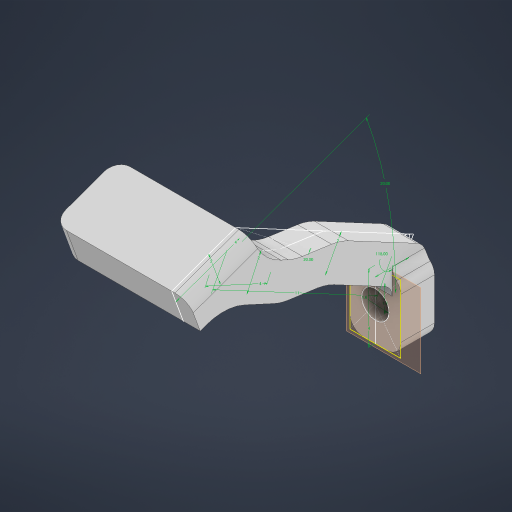
# Autodesk Inventor part: battery-stopper-1
Saved by Autodesk Inventor 2023.5 (Build 275446000, 446)
## iProperties
Created: 2025-02-09
Part Number: battery-stopper-1
Material: 一般
Document SubType Name: Modeling
Designer: IshiiLabHonda
Density: 1 g/cm^3
Appearance: 既定
Author: IshiiLabHonda
Autodesk Inventor part; units mm, degrees
ref_plane "YZ Plane" through (0, 0, 0) normal (1, 0, 0) x (0, 1, 0)
ref_plane "XZ Plane" through (0, 0, 0) normal (0, 1, 0) x (-1, 0, 0)
ref_plane "XY Plane" through (0, 0, 0) normal (0, 0, 1) x (1, 0, 0)
sketch "スケッチ5" plane through (0, 0, 0) normal (1, 0, 0) x (0, 1, 0)
  line L0 (0, 0) -> (0, 1.293622) construction
  line L1 (0, 0) -> (-1.333849, 0) construction
  line L2 (2, 2) -> (-2, 2)
  line L3 (-2, 2) -> (-2, 0)
  line L4 (-2, 0) -> (2, 0)
  line L5 (2, 0) -> (2, 2)
  line L6 (0.8, 2) -> (0.8, 0)
  line L7 (-0.8, 2) -> (-0.8, 0)
  line L8 (-2, 1) -> (2, 1) construction
  line L9 (2, 1) -> (7.164187, 10.712424) construction
  line L10 (8.047135, 10.242952) -> (6.28124, 11.181895)
  line L11 (6.28124, 11.181895) -> (0.702534, 0.689875)
  line L12 (0.702534, 0.689875) -> (2.468429, -0.249068)
  line L13 (2.468429, -0.249068) -> (8.047135, 10.242952)
  line L14 (2, 0) -> (2.600861, 0)
  line L15 (6.679054, 14.001722) -> (4.799669, 13.317682)
  line L16 (4.799669, 13.317682) -> (6.16775, 9.558912)
  line L17 (6.16775, 9.558912) -> (8.047135, 10.242952)
  line L18 (8.047135, 10.242952) -> (6.679054, 14.001722)
  line L19 (6.679054, 14.001722) -> (6.16775, 9.558912) construction
  line L20 (4.799669, 13.317682) -> (8.047135, 10.242952) construction
  line L21 (5.739362, 13.659702) -> (7.107442, 9.900932) construction
  line L22 (6.423402, 11.780317) -> (4.751494, 8.146487) construction
  line L23 (4.751494, 8.146487) -> (4.374834, 5.466414) construction
  line L24 (6.28124, 11.181895) -> (2.468429, -0.249068) construction
  line L25 (0.702534, 0.689875) -> (8.047135, 10.242952) construction
  line L26 (7.331859, 11.36234) -> (5.514944, 12.198294)
  line L27 (5.514944, 12.198294) -> (3.843036, 8.564464)
  line L28 (3.843036, 8.564464) -> (5.659952, 7.72851)
  line L29 (5.659952, 7.72851) -> (7.331859, 11.36234)
  line L30 (7.331859, 11.36234) -> (3.843036, 8.564464) construction
  line L31 (5.514944, 12.198294) -> (5.659952, 7.72851) construction
  line L32 (5.659952, 7.72851) -> (5.28262, 5.043656)
  line L33 (3.843036, 8.564464) -> (2.653219, 0.098471)
  line L34 (3.467048, 5.889171) -> (5.232944, 4.950228)
  point P0 (1.399139, 2)
  point P1 (5.587448, 9.963402)
  point P2 (5.343064, 11.824718)
  point P3 (6.569366, 9.705088)
  dimension "d25" = 1.6
  dimension "d26" = 4
  dimension "d27" = 2
  dimension "d28" = 118
  dimension "d29" = 2
  dimension "d30" = 11
  dimension "d44" = 2
  dimension "d45" = 20
  dimension "d46" = 4
  dimension "d52" = 20
  dimension "d53" = 4
  dimension "d54" = 2
  constraints: 70 end point, 15 midpoint, 15 point on line, 10 parallel, 7 perpendicular, 1 coincident, 1 vertical, 6 other
  measures "d25" distance between parallel lines of L7 L6
  measures "d26" distance between parallel lines of L3 L5
  measures "d27" distance between parallel lines of L4 L2
  measures "d28" angle of L8 L9
  measures "d29" distance between parallel lines of L13 L11
  measures "d30" distance of L8.end L9.end
  measures "d44" distance between parallel lines of L18 L16
  measures "d45" angle of L0 L21
  measures "d46" distance between parallel lines of L17 L15
  measures "d52" angle of L9 L23
  measures "d53" distance of L22.start L22.end
  measures "d54" distance between parallel lines of L29 L27
extrude "押し出し8" add sketch "スケッチ5" along normal mid plane 3 contours L6 L11 L12 L4 L7 L2 | L2 L11 L6 | L7 L4 L3 L2 | L2 L5 L12 L6 L11 | L6 L12 L11 | L12 L4 L6
ref_plane "作業平面7" through (-1.5, -2, 2) normal (0, 0, 1) x (1, 0, 0)
sketch "スケッチ6" plane through (-1.5, -2, 2) normal (0, 0, 1) x (1, 0, 0)
  line L0 (3, 0) -> (0, 0) projected
  line L1 (3, 4) -> (3, 0) projected
  line L2 (0, 4) -> (3, 4) projected
  line L3 (0, 0) -> (0, 4) projected
  line L4 (0, 4) -> (3, 4) projected
  line L5 (0, 4) -> (3, 0) construction
  line L6 (0, 0) -> (3, 0) projected
  line L7 (3, 0) -> (3, 4) projected
  line L8 (0, 0) -> (3, 4) construction
  circle A0 centre (1.5, 2) radius 0.8
  dimension "d35" = 1.6
  constraints: 4 end point, 1 centre point, 1 coincident
  measures "d35" diameter of A0
extrude "押し出し9" cut sketch "スケッチ6" against normal blind 4 contours A0
extrude "押し出し13" add sketch "スケッチ5" along normal blind 7 contours L16 L27 L26 L29 L10 L11 | L11 L10 L29 L17 L16 | L16 L15 L18 L10 L29 L26 L27 | L29 L10 L17
extrude "押し出し15" add sketch "スケッチ5" along normal mid plane 2 contours L11 L33 L13 L14 L5 L2 | L33 L28 L11 | L34 L13 L33 | L11 L28 L32 L13 L34 | L28 L27 L16 L11 | L11 L16 L17 L29 L28 | L16 L27 L26 L29 L10 L11 | L11 L10 L29 L17 L16
extrude "押し出し16" add sketch "スケッチ5" against normal blind 1 contours L16 L15 L18 L10 L29 L26 L27 | L29 L10 L17
fillet "フィレット1" radius 0.8 1 edges at (0, 1.3991, 2)
fillet "フィレット2" radius 1 1 edges at (0, 2.6009, 0)
fillet "フィレット3" radius 3 4 edges at (0, 5.2826, 5.0437) (0, 3.467, 5.8892) (0, 3.843, 8.5645) (0, 5.66, 7.7285)
fillet "フィレット4" radius 3 2 edges at (0, 5.3431, 11.8247) (0, 6.5694, 9.7051)
fillet "フィレット5" radius 0.8 8 edges at (7, 5.7394, 13.6597) (7, 7.1074, 9.9009) (-1.5, -2, 1) (-1.5, 2, 1) (1.5, 2, 1) (1.5, -2, 1) (1, 2, 1) (-1, 2, 1)
fillet "フィレット6" radius 0.8 1 edges at (-1, 7.3631, 12.1223)
mirror "ミラー1" about plane through (0, 0, 0) normal (1, 0, 0) remove original yes
fillet "フィレット7" radius 0.4 1 edges at (-1, 5.5444, 11.2714)
